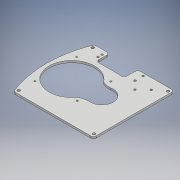
# Autodesk Inventor part: 06-01-Платформа для лидара
Saved by Autodesk Inventor 2018 (Build 220112000, 112)
## iProperties
Created: 2018-12-15
Part Number: 06-01-Платформа для лидара
Material: Типовые
Document SubType Name: Modeling
Designer: RR
Density: 1 g/cm^3
Appearance: По умолчанию
Author: RR
Autodesk Inventor part; units mm, degrees
ref_plane "YZ Plane" through (0, 0, 0) normal (1, 0, 0) x (0, 1, 0)
ref_plane "XZ Plane" through (0, 0, 0) normal (0, 1, 0) x (-1, 0, 0)
ref_plane "XY Plane" through (0, 0, 0) normal (0, 0, 1) x (1, 0, 0)
sketch "Эскиз1" plane through (0, 0, 0) normal (0, 0, 1) x (1, 0, 0)
  line L0 (0, 29) -> (0, -30)
  circle A0 centre (35, 25) radius 1.25
  circle A1 centre (-22, 31) radius 1.25
  circle A2 centre (-22, -31) radius 1.25
  circle A3 centre (35, -25) radius 1.25
  arc A4 (45.1579, -16.824) -> (42.7931, 16.7046) centre (46.5307, 0.1205) ccw
  line L1 (35, -25) -> (0, -25)
  circle A5 centre (-22, -55) radius 2
  circle A6 centre (90, -55) radius 2
  circle A7 centre (90, 55) radius 2
  circle A8 centre (-22, 55) radius 2
  line L2 (-22, -60) -> (90, -60)
  line L3 (94, -56) -> (94, 56)
  arc A9 (94, 56) -> (90, 60) centre (90, 56) ccw
  arc A10 (90, -60) -> (94, -56) centre (90, -56) ccw
  arc A11 (-24.8284, -58.8284) -> (-22, -60) centre (-22, -56) ccw
  arc A12 (-22, 60) -> (-24.8284, 58.8284) centre (-22, 56) ccw
  line L4 (94, 0) -> (94, 6)
  circle A13 centre (52, 44) radius 1.5
  circle A14 centre (52, 56) radius 1.5
  line L5 (-22, 60) -> (-6, 60)
  line L6 (44, 60) -> (90, 60)
  arc A15 (46.5295, -16.8795) -> (30.2933, -20.5081) centre (44.6409, -46.5678) ccw
  arc A16 (30.2933, 18.9458) -> (42.7931, 16.7046) centre (41.489, 45.4087) ccw
  line L7 (36, 40) -> (2, 40)
  line L8 (-2, 44) -> (-2, 56)
  line L9 (40, 56) -> (40, 44)
  arc A17 (44, 60) -> (40, 56) centre (44, 56) ccw
  arc A18 (36, 40) -> (40, 44) centre (36, 44) ccw
  arc A19 (-2, 44) -> (2, 40) centre (2, 44) ccw
  arc A20 (-2, 56) -> (-6, 60) centre (-6, 56) ccw
  circle A21 centre (-6, 53) radius 1.5
  circle A22 centre (-6, 47) radius 1.5
  arc A23 (-24.8284, 58.8284) -> (-24.8284, -58.8284) centre (124.4782, 0) ccw
  circle A24 centre (63.4885, 32.25) radius 1.5
  circle A25 centre (76, 44) radius 1.5
  arc A26 (30.2933, 18.9458) -> (30.2933, -20.5081) centre (2.8162, -0.7812) ccw
  point P0 (0, 0)
  point P1 (-26, -60)
  point P2 (94, -60)
  dimension "d3" = 2.5
  dimension "d4" = 2.5
  dimension "d5" = 2.5
  dimension "d6" = 2.5
  dimension "d10" = 50
  dimension "d11" = 34
  dimension "d39" = 4
  dimension "d44" = 120
  dimension "d46" = 4
  dimension "d70" = 4
  dimension "d71" = 3
  dimension "d72" = 3
  dimension "d75" = 3
  dimension "d76" = 3
  constraints: 28 point on circle, 27 centre point, 20 end point, 13 tangent, 6 equal radius, 5 point on line, 3 perpendicular, 2 vertical, 1 collinear, 1 horizontal, 1 midpoint
  measures "d3" diameter of A0
  measures "d4" diameter of A1
  measures "d5" diameter of A2
  measures "d6" diameter of A3
  measures "d10" distance of L1.start A0.centre
  measures "d11" diameter of A4
  measures "d39" diameter of A7
  measures "d44" distance of point (-26, -60) point (94, -60)
  measures "d46" radius of A9
  measures "d70" radius of A17
  measures "d71" diameter of A21
  measures "d72" diameter of A22
  measures "d75" diameter of A24
  measures "d76" diameter of A25
extrude "Выдавливание4" add sketch "Эскиз1" along normal blind 3
